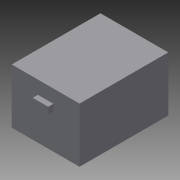
# Autodesk Inventor part: s0.57A 10V Diode
Saved by Autodesk Inventor 2015 (Build 190159000, 159)
## iProperties
Created: 2016-01-19
Part Number: s0.57A 10V Diode
Material: Generic
Document SubType Name: Modeling
Designer: Kyle
Density: 1 g/cm^3
Appearance: Default
Author: Kyle
Autodesk Inventor part; units mm, degrees
ref_plane "YZ Plane" through (0, 0, 0) normal (1, 0, 0) x (0, 1, 0)
ref_plane "XZ Plane" through (0, 0, 0) normal (0, 1, 0) x (-1, 0, 0)
ref_plane "XY Plane" through (0, 0, 0) normal (0, 0, 1) x (1, 0, 0)
sketch "Sketch1" plane through (0, 0, 0) normal (0, 0, 1) x (1, 0, 0)
  line L0 (0, 0) -> (1.3005, 0)
  line L1 (1.3005, 0) -> (1.3005, 1.049)
  line L2 (1.3005, 1.049) -> (0, 1.049)
  line L3 (0, 1.049) -> (0, 0)
  dimension "d0" = 1.049
  dimension "d1" = 1.3005
  constraints: 8 end point, 2 parallel, 1 horizontal, 1 perpendicular
  measures "d0" distance of L0.end L1.end
  measures "d1" distance of L1.end L2.end
extrude "Extrusion1" add sketch "Sketch1" along normal blind 1.7018
sketch "Sketch2" plane through (0, 0, 1.7018) normal (0, 0, 1) x (1, 0, 0)
  line L0 (0.5004, 0.795) -> (0.8001, 0.795)
  line L1 (0.8001, 0.795) -> (0.8001, 0.6706)
  line L2 (0.8001, 0.6706) -> (0.5004, 0.6706)
  line L3 (0.5004, 0.6706) -> (0.5004, 0.795)
  line L4 (0, 1.049) -> (0, 0) projected
  line L5 (1.3005, 1.049) -> (0, 1.049) projected
  dimension "d4" = 0.2997
  dimension "d5" = 0.5004
  dimension "d6" = 0.254
  dimension "d7" = 0.1245
  constraints: 8 end point, 2 parallel, 1 horizontal, 1 perpendicular
  measures "d4" distance of L0.start L0.end
  measures "d5" distance between parallel lines of L4 L3
  measures "d6" distance between parallel lines of L5 L0
  measures "d7" distance between parallel lines of L0 L2
extrude "Extrusion2" add sketch "Sketch2" against normal blind 1.8009
extrude "Extrusion3" add sketch "Sketch2" along normal blind 0.0991
body "Solid1"
